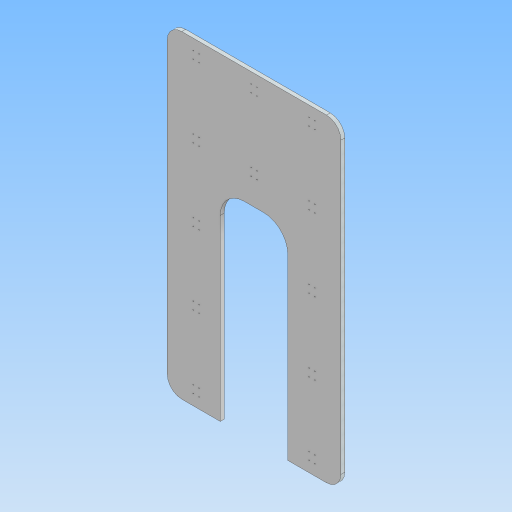
# Autodesk Inventor part: Wagen_Platte
Saved by Autodesk Inventor 2024.4 (Build 284460000, 460)
## iProperties
Created: 2026-01-22
Part Number: Wagen_Platte
Material: Generisch
Document SubType Name: Modeling
Designer: windows-desktop
Mass: 47117.4 g
Surface Area: 188463 cm^2
Volume: 47117.4 cm^3
Density: 1 g/cm^3
Appearance: Vorgabe
Masse[kg]: 47,1 kg
Autodesk Inventor part; units mm, degrees
ref_plane "YZ Plane" through (0, 0, 0) normal (1, 0, 0) x (0, 1, 0)
ref_plane "XZ Plane" through (0, 0, 0) normal (0, 1, 0) x (-1, 0, 0)
ref_plane "XY Plane" through (0, 0, 0) normal (0, 0, 1) x (1, 0, 0)
sketch "Skizze1" plane through (0, 0, 0) normal (0, 1, 0) x (-1, 0, 0)
  line L0 (1211.3292, 1483.4558) -> (-288.6708, 1483.4558)
  line L1 (-438.6708, 1333.4558) -> (-438.6708, -1666.5442)
  line L2 (-288.6708, -1816.5442) -> (1211.3292, -1816.5442)
  line L3 (1361.3292, -1666.5442) -> (1361.3292, 1333.4558)
  arc A0 (1211.3292, -1816.5442) -> (1361.3292, -1666.5442) centre (1211.3292, -1666.5442) ccw
  arc A1 (1361.3292, 1333.4558) -> (1211.3292, 1483.4558) centre (1211.3292, 1333.4558) ccw
  arc A2 (-288.6708, 1483.4558) -> (-438.6708, 1333.4558) centre (-288.6708, 1333.4558) ccw
  arc A3 (-438.6708, -1666.5442) -> (-288.6708, -1816.5442) centre (-288.6708, -1666.5442) ccw
  point P0 (0, 0)
  point P1 (1361.3292, 1483.4558)
  point P2 (-438.6708, -1816.5442)
  point P3 (1361.3292, -1816.5442)
  dimension "d0" = 1800
  dimension "d1" = 3300
  dimension "d2" = 150
  dimension "d3" = 150
  constraints: 8 end point, 8 point on circle, 8 tangent, 6 point on line, 4 centre point, 2 equal radius, 2 parallel, 1 horizontal, 1 perpendicular
  measures "d0" distance of point (-438.671, -1816.544) point (1361.329, -1816.544)
  measures "d1" distance of point (1361.329, -1816.544) point (1361.329, 1483.456)
  measures "d2" radius of A0
  measures "d3" radius of A1
extrude "Extrusion1" add sketch "Skizze1" along normal blind 40
sketch "Skizze3" plane through (0, 0, 0) normal (0, -1, 0) x (1, 0, 0)
  circle A0 centre (-1031.3292, 1294.2058) radius 2.4585 construction
  circle A1 centre (-1091.3292, 1294.2058) radius 2.4585 construction
  circle A2 centre (-1091.3292, 1372.7058) radius 2.4585 construction
  circle A3 centre (-1031.3292, 1372.7058) radius 2.4585 construction
  circle A4 centre (168.6708, -1627.2942) radius 2.4585 construction
  circle A5 centre (108.6708, -1627.2942) radius 2.4585 construction
  circle A6 centre (108.6708, -1705.7942) radius 2.4585 construction
  circle A7 centre (168.6708, -1705.7942) radius 2.4585 construction
  circle A8 centre (-431.3292, -1627.2942) radius 2.4585 construction
  circle A9 centre (-491.3292, -1627.2942) radius 2.4585 construction
  circle A10 centre (-491.3292, -1705.7942) radius 2.4585 construction
  circle A11 centre (-431.3292, -1705.7942) radius 2.4585 construction
  circle A12 centre (-1091.3292, -1627.2942) radius 2.4585 construction
  circle A13 centre (-1031.3292, -1627.2942) radius 2.4585 construction
  circle A14 centre (-1091.3292, -1705.7942) radius 2.4585 construction
  circle A15 centre (-1031.3292, -1705.7942) radius 2.4585 construction
  circle A16 centre (168.6708, -877.2942) radius 2.4585 construction
  circle A17 centre (108.6708, -877.2942) radius 2.4585 construction
  circle A18 centre (108.6708, -955.7942) radius 2.4585 construction
  circle A19 centre (168.6708, -955.7942) radius 2.4585 construction
  circle A20 centre (-431.3292, -877.2942) radius 2.4585 construction
  circle A21 centre (-491.3292, -877.2942) radius 2.4585 construction
  circle A22 centre (-491.3292, -955.7942) radius 2.4585 construction
  circle A23 centre (-431.3292, -955.7942) radius 2.4585 construction
  circle A24 centre (-1091.3292, -877.2942) radius 2.4585 construction
  circle A25 centre (-1031.3292, -877.2942) radius 2.4585 construction
  circle A26 centre (-1091.3292, -955.7942) radius 2.4585 construction
  circle A27 centre (-1031.3292, -955.7942) radius 2.4585 construction
  circle A28 centre (168.6708, -127.2942) radius 2.4585 construction
  circle A29 centre (108.6708, -127.2942) radius 2.4585 construction
  circle A30 centre (108.6708, -205.7942) radius 2.4585 construction
  circle A31 centre (168.6708, -205.7942) radius 2.4585 construction
  circle A32 centre (-431.3292, -127.2942) radius 2.4585 construction
  circle A33 centre (-491.3292, -127.2942) radius 2.4585 construction
  circle A34 centre (-491.3292, -205.7942) radius 2.4585 construction
  circle A35 centre (-431.3292, -205.7942) radius 2.4585 construction
  circle A36 centre (-1091.3292, -127.2942) radius 2.4585 construction
  circle A37 centre (-1031.3292, -127.2942) radius 2.4585 construction
  circle A38 centre (-1091.3292, -205.7942) radius 2.4585 construction
  circle A39 centre (-1031.3292, -205.7942) radius 2.4585 construction
  circle A40 centre (168.6708, 622.7058) radius 2.4585 construction
  circle A41 centre (108.6708, 622.7058) radius 2.4585 construction
  circle A42 centre (108.6708, 544.2058) radius 2.4585 construction
  circle A43 centre (168.6708, 544.2058) radius 2.4585 construction
  circle A44 centre (-431.3292, 622.7058) radius 2.4585 construction
  circle A45 centre (-491.3292, 622.7058) radius 2.4585 construction
  circle A46 centre (-491.3292, 544.2058) radius 2.4585 construction
  circle A47 centre (-431.3292, 544.2058) radius 2.4585 construction
  circle A48 centre (-1091.3292, 622.7058) radius 2.4585 construction
  circle A49 centre (-1031.3292, 622.7058) radius 2.4585 construction
  circle A50 centre (-1091.3292, 544.2058) radius 2.4585 construction
  circle A51 centre (-1031.3292, 544.2058) radius 2.4585 construction
  circle A52 centre (168.6708, 1294.2058) radius 2.4585 construction
  circle A53 centre (108.6708, 1294.2058) radius 2.4585 construction
  circle A54 centre (-431.3292, 1294.2058) radius 2.4585 construction
  circle A55 centre (-491.3292, 1294.2058) radius 2.4585 construction
  circle A56 centre (108.6708, 1372.7058) radius 2.4585 construction
  circle A57 centre (168.6708, 1372.7058) radius 2.4585 construction
  circle A58 centre (-491.3292, 1372.7058) radius 2.4585 construction
  circle A59 centre (-431.3292, 1372.7058) radius 2.4585 construction
  line L0 (288.6708, -1816.5442) -> (-1211.3292, -1816.5442) construction
  line L1 (-461.3292, -1816.5442) -> (-461.3292, 283.4558)
  line L2 (-461.3292, -1816.5442) -> (-111.3292, -1816.5442)
  line L3 (-461.3292, 1333.4558) -> (-461.3292, 283.4558)
  line L4 (-461.3292, 1333.4558) -> (138.6708, 1333.4558)
  line L5 (-461.3292, 1333.4558) -> (-1061.3292, 1333.4558)
  line L6 (-461.3292, -1816.5442) -> (-811.3292, -1816.5442)
  line L7 (-111.3292, -1816.5442) -> (-811.3292, -1816.5442)
  line L8 (-111.3292, -1816.5442) -> (-811.3292, -1816.5442)
  line L9 (-811.3292, -1816.5442) -> (-811.3292, 33.4558)
  line L10 (-561.3292, 283.4558) -> (-361.3292, 283.4558)
  line L11 (-111.3292, 33.4558) -> (-111.3292, -1816.5442)
  arc A60 (-561.3292, 283.4558) -> (-811.3292, 33.4558) centre (-561.3292, 33.4558) ccw
  arc A61 (-111.3292, 33.4558) -> (-361.3292, 283.4558) centre (-361.3292, 33.4558) ccw
  point P0 (0, 0)
  dimension "d43" = 2100
  dimension "d44" = 350
  dimension "d45" = 600
  dimension "d46" = 600
  dimension "d47" = 350
  dimension "d48" = 250
  constraints: 22 end point, 4 point on circle, 4 tangent, 3 horizontal, 2 centre point, 2 parallel, 2 perpendicular, 2 point on line, 2 vertical, 1 equal radius, 1 midpoint
  measures "d43" distance of L1.start L1.end
  measures "d44" distance of L1.start L2.end
  measures "d45" distance of L3.start L4.end
  measures "d46" distance of L3.start L5.end
  measures "d47" distance of L1.start L6.end
  measures "d48" radius of A60
extrude "Extrusion2" cut sketch "Skizze3" against normal through all
hole "Bohrung2" at (-1091.3292, 0, -1627.2942) at (-1091.3292, 0, -1705.7942) at (-1031.3292, 0, -1627.2942) at (-1031.3292, 0, -1705.7942) at (-1091.3292, 0, -877.2942) at (-1031.3292, 0, -877.2942) at (-1031.3292, 0, -955.7942) at (-1091.3292, 0, -955.7942) at (-1091.3292, 0, -127.2942) at (-1031.3292, 0, -127.2942) at (-1031.3292, 0, -205.7942) at (-1091.3292, 0, -205.7942) at (108.6708, 0, -1627.2942) at (168.6708, 0, -1627.2942) at (108.6708, 0, -1705.7942) at (168.6708, 0, -1705.7942) at (108.6708, 0, -877.2942) at (168.6708, 0, -877.2942) at (168.6708, 0, -955.7942) at (108.6708, 0, -955.7942) at (108.6708, 0, -127.2942) at (168.6708, 0, -127.2942) at (168.6708, 0, -205.7942) at (108.6708, 0, -205.7942) at (-1091.3292, 0, 622.7058) at (-1031.3292, 0, 622.7058) at (-1031.3292, 0, 544.2058) at (-1091.3292, 0, 544.2058) at (-491.3292, 0, 622.7058) at (-431.3292, 0, 622.7058) at (-431.3292, 0, 544.2058) at (-491.3292, 0, 544.2058) at (108.6708, 0, 622.7058) at (168.6708, 0, 622.7058) at (168.6708, 0, 544.2058) at (108.6708, 0, 544.2058) at (-1091.3292, 0, 1372.7058) at (-1031.3292, 0, 1372.7058) at (-1031.3292, 0, 1294.2058) at (-1091.3292, 0, 1294.2058) at (-491.3292, 0, 1372.7058) at (-431.3292, 0, 1372.7058) at (-431.3292, 0, 1294.2058) at (-491.3292, 0, 1294.2058) at (108.6708, 0, 1372.7058) at (168.6708, 0, 1372.7058) at (168.6708, 0, 1294.2058) at (108.6708, 0, 1294.2058) direction (0, 1, 0) diameter 8.376 depth 26 tip angle 118 thread size "M10x1.5" class "6H" standard "ISO Metric profile"
shell "Wandung1" thickness 5 removed faces 0
